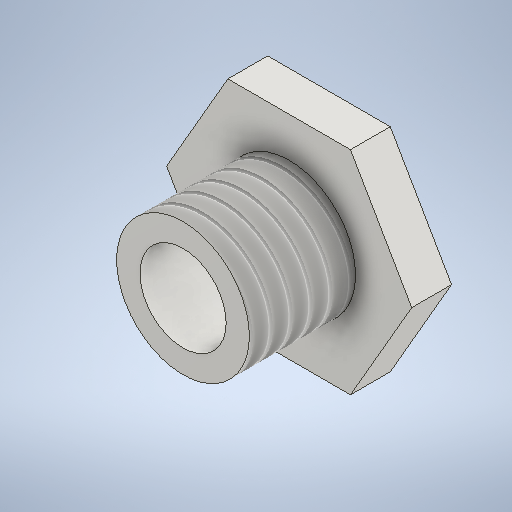
# Autodesk Inventor part: 10a GLAND NUT
Saved by Autodesk Inventor 2025.2 (Build 292293000, 293)
## iProperties
Created: 2025-06-19
Part Number: 10a GLAND NUT
Material: Steel AISI 1020 107 HR
Document SubType Name: Modeling
Designer: bless
Density: 7.87 g/cm^3
Appearance: Steel
Author: bless
Autodesk Inventor part; units mm, degrees
ref_plane "YZ Plane" through (0, 0, 0) normal (1, 0, 0) x (0, 1, 0)
ref_plane "XZ Plane" through (0, 0, 0) normal (0, 1, 0) x (-1, 0, 0)
ref_plane "XY Plane" through (0, 0, 0) normal (0, 0, 1) x (1, 0, 0)
sketch "Sketch1" plane through (0, 0, 0) normal (0, 0, 1) x (1, 0, 0)
  line L0 (9.2376, 0) -> (4.6188, -8)
  line L1 (4.6188, -8) -> (-4.6188, -8)
  line L2 (-4.6188, -8) -> (-9.2376, 0)
  line L3 (-9.2376, 0) -> (-4.6188, 8)
  line L4 (-4.6188, 8) -> (4.6188, 8)
  line L5 (4.6188, 8) -> (9.2376, 0)
  point P0 (0, 0)
  point P1 (0, 0)
  dimension "d0" = 16
  constraints: 12 end point, 1 coincident, 1 horizontal, 13 other
  measures "d0" distance between parallel lines of L1 L4
extrude "Extrusion1" add sketch "Sketch1" along normal blind 3
sketch "Sketch2" plane through (0, 0, 3) normal (0, 0, 1) x (1, 0, 0)
  circle A0 centre (0, 0) radius 5
  dimension "d3" = 10
  constraints: 1 centre point, 1 coincident
  measures "d3" diameter of A0
extrude "Extrusion2" add sketch "Sketch2" along normal blind 8
sketch "Sketch3" plane through (0, 0, 11) normal (0, 0, 1) x (1, 0, 0)
  circle A0 centre (0, 0) radius 5 projected
  constraints: 1 coincident
hole "Hole1" at (0, 0, 11) direction (0, 0, -1) diameter 6.5 end through all
thread "Thread1" size "M10x1.5" class "6g" standard "ANSI Metric M Profile" length 8
body "Solid1"
